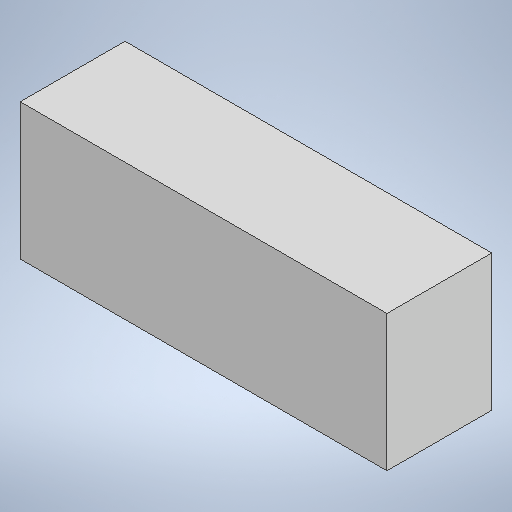
# Autodesk Inventor part: Leitstange sicherungsblock 001
Saved by Autodesk Inventor 2025 (Build 290162000, 162)
## iProperties
Created: 2024-04-08
Part Number: Leitstange sicherungsblock 001
Material: Generisch
Document SubType Name: Modeling
Designer: noahm
Density: 1 g/cm^3
Appearance: Vorgabe
Author: noahm
Autodesk Inventor part; units mm, degrees
ref_plane "YZ Plane" through (0, 0, 0) normal (1, 0, 0) x (0, 1, 0)
ref_plane "XZ Plane" through (0, 0, 0) normal (0, 1, 0) x (-1, 0, 0)
ref_plane "XY Plane" through (0, 0, 0) normal (0, 0, 1) x (1, 0, 0)
sketch "Skizze1" plane through (0, 0, 0) normal (0, 1, 0) x (-1, 0, 0)
  line L0 (-8.75, -3.25) -> (8.75, -3.25)
  line L1 (8.75, -3.25) -> (8.75, 3.25)
  line L2 (8.75, 3.25) -> (-8.75, 3.25)
  line L3 (-8.75, 3.25) -> (-8.75, -3.25)
  line L4 (-8.75, -3.25) -> (8.75, 3.25) construction
  line L5 (8.75, -3.25) -> (-8.75, 3.25) construction
  point P0 (0, 0)
  dimension "d0" = 6.5
  dimension "d1" = 17.5
  constraints: 12 end point, 2 midpoint, 2 parallel, 1 horizontal, 1 perpendicular
  measures "d0" distance of L0.end L1.end
  measures "d1" distance of L1.end L2.end
extrude "Extrusion1" add sketch "Skizze1" along normal blind 5
